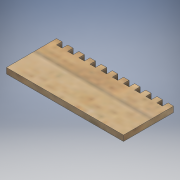
# Autodesk Inventor part: Side Support
Saved by Autodesk Inventor 2017 (Build 210142000, 142)
## iProperties
Created: 2017-05-02
Part Number: Side Support
Material: Generic
Document SubType Name: Modeling
Designer: Parshant Bombhi
Density: 1 g/cm^3
Appearance: Natural Maple - Glossy Dark Tint
Author: Parshant Bombhi
Autodesk Inventor part; units mm, degrees
ref_plane "YZ Plane" through (0, 0, 0) normal (1, 0, 0) x (0, 1, 0)
ref_plane "XZ Plane" through (0, 0, 0) normal (0, 1, 0) x (-1, 0, 0)
ref_plane "XY Plane" through (0, 0, 0) normal (0, 0, 1) x (1, 0, 0)
sketch "Sketch2" plane through (0, 0, 0) normal (0, 0, 1) x (1, 0, 0)
  line L0 (0, 0) -> (133.35, 0)
  line L1 (133.35, 0) -> (133.35, 57.15)
  line L2 (0, 57.15) -> (0, 0)
  line L3 (0, 57.15) -> (6.35, 57.15)
  line L4 (6.35, 57.15) -> (6.35, 50.8)
  line L5 (6.35, 50.8) -> (12.7, 50.8)
  line L6 (12.7, 50.8) -> (12.7, 57.15)
  line L7 (12.7, 57.15) -> (19.05, 57.15)
  line L8 (19.05, 57.15) -> (19.05, 50.8)
  line L9 (19.05, 50.8) -> (25.4, 50.8)
  line L10 (25.4, 50.8) -> (25.4, 57.15)
  line L11 (25.4, 57.15) -> (31.75, 57.15)
  line L12 (31.75, 57.15) -> (31.75, 50.8)
  line L13 (31.75, 50.8) -> (38.1, 50.8)
  line L14 (38.1, 50.8) -> (38.1, 57.15)
  line L15 (38.1, 57.15) -> (44.45, 57.15)
  line L16 (44.45, 57.15) -> (44.45, 50.8)
  line L17 (44.45, 50.8) -> (50.8, 50.8)
  line L18 (50.8, 50.8) -> (50.8, 57.15)
  line L19 (50.8, 57.15) -> (57.15, 57.15)
  line L20 (57.15, 57.15) -> (57.15, 50.8)
  line L21 (57.15, 50.8) -> (63.5, 50.8)
  line L22 (63.5, 50.8) -> (63.5, 57.15)
  line L23 (63.5, 57.15) -> (69.85, 57.15)
  line L24 (69.85, 57.15) -> (69.85, 50.8)
  line L25 (69.85, 50.8) -> (76.2, 50.8)
  line L26 (76.2, 50.8) -> (76.2, 57.15)
  line L27 (76.2, 57.15) -> (82.55, 57.15)
  line L28 (82.55, 57.15) -> (82.55, 50.8)
  line L29 (82.55, 50.8) -> (88.9, 50.8)
  line L30 (88.9, 50.8) -> (88.9, 57.15)
  line L31 (88.9, 57.15) -> (95.25, 57.15)
  line L32 (95.25, 57.15) -> (95.25, 50.8)
  line L33 (95.25, 50.8) -> (101.6, 50.8)
  line L34 (101.6, 50.8) -> (101.6, 57.15)
  line L35 (101.6, 57.15) -> (107.95, 57.15)
  line L36 (107.95, 57.15) -> (107.95, 50.8)
  line L37 (107.95, 50.8) -> (114.3, 50.8)
  line L38 (114.3, 50.8) -> (114.3, 57.15)
  line L39 (114.3, 57.15) -> (120.65, 57.15)
  line L40 (120.65, 57.15) -> (120.65, 50.8)
  line L41 (120.65, 50.8) -> (127, 50.8)
  line L42 (127, 50.8) -> (127, 57.15)
  line L43 (127, 57.15) -> (133.35, 57.15)
  dimension "Length" = 133.35
  dimension "Height" = 57.15
  dimension "Teeth_Width" = 6.35
  dimension "Material_Thickness" = 6.35
  dimension "d63" = 6.35
  dimension "d64" = 6.35
  dimension "d65" = 6.35
  dimension "d66" = 6.35
  dimension "d67" = 6.35
  dimension "d68" = 6.35
  dimension "d69" = 6.35
  dimension "d70" = 6.35
  dimension "d71" = 6.35
  dimension "d72" = 6.35
  dimension "d73" = 6.35
  dimension "d74" = 6.35
  dimension "d75" = 6.35
  dimension "d76" = 6.35
  dimension "d77" = 6.35
  dimension "d78" = 6.35
  dimension "d79" = 6.35
  dimension "d80" = 6.35
  dimension "d81" = 6.35
  dimension "d82" = 6.35
  dimension "d83" = 6.35
  dimension "d84" = 6.35
  dimension "d85" = 6.35
  dimension "d86" = 6.35
  dimension "d87" = 6.35
  dimension "d88" = 6.35
  dimension "d89" = 6.35
  dimension "d90" = 6.35
  constraints: 88 end point, 31 perpendicular, 12 horizontal, 10 point on line, 1 parallel
  measures "Length" distance of L0.start L0.end
  measures "Height" distance of L2.start L0.start
  measures "Teeth_Width" distance of L2.start L3.end
  measures "Material_Thickness" distance of L3.end L4.end
  measures "d63" distance of L4.end L5.end
  measures "d64" distance of L6.end L8.start
  measures "d65" distance of L8.start L9.start
  measures "d66" distance of L9.start L10.start
  measures "d67" distance of L10.end L12.start
  measures "d68" distance of L12.start L13.start
  measures "d69" distance of L13.start L14.start
  measures "d70" distance of L14.end L16.start
  measures "d71" distance of L16.start L17.start
  measures "d72" distance of L17.start L18.start
  measures "d73" distance of L18.end L20.start
  measures "d74" distance of L20.start L21.start
  measures "d75" distance of L21.start L22.start
  measures "d76" distance of L22.end L24.start
  measures "d77" distance of L24.start L25.start
  measures "d78" distance of L25.start L26.start
  measures "d79" distance of L26.end L28.start
  measures "d80" distance of L28.start L29.start
  measures "d81" distance of L29.start L30.start
  measures "d82" distance of L30.end L32.start
  measures "d83" distance of L32.start L33.start
  measures "d84" distance of L33.start L34.start
  measures "d85" distance of L34.end L36.start
  measures "d86" distance of L36.start L37.start
  measures "d87" distance of L37.start L38.start
  measures "d88" distance of L38.end L40.start
  measures "d89" distance of L40.start L41.start
  measures "d90" distance of L41.start L42.start
extrude "Extrusion2" add sketch "Sketch2" along normal blind 6.35
equation "\"d63\" = Teeth_Width"
equation "\"d66\" = d64"
equation "\"d69\" = d67"
equation "\"d72\" = d70"
equation "\"d75\" = d73"
equation "\"d78\" = d76"
equation "\"d81\" = d79"
equation "\"d84\" = d82"
equation "\"d87\" = d85"
equation "\"d90\" = d88"
body "Solid2"
